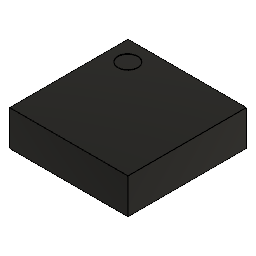
IMU v1 (Autodesk Fusion 360 design; units mm, degrees)
Autodesk Fusion 360 part; units mm, degrees
sketch "スケッチ1" plane through (0, 0, 0) normal (0, 0, 1) x (1, 0, 0)
  line L0 (1.5, 1.5) -> (-1.5, 1.5)
  line L1 (-1.5, 1.5) -> (-1.5, -1.5)
  line L2 (-1.5, -1.5) -> (1.5, -1.5)
  line L3 (1.5, -1.5) -> (1.5, 1.5)
  line L4 (1.5, 1.5) -> (-1.5, -1.5) construction
  line L5 (-1.5, 1.5) -> (1.5, -1.5) construction
  dimension "d1" = 3
  dimension "d2" = 3
extrude "押し出し1" add sketch "スケッチ1" along normal blind 0.9
sketch "スケッチ2" plane through (0, 0, 0.9) normal (0, 0, 1) x (-1, 0, 0)
  line L0 (-1.5, 1.5) -> (-1.5, -1.5)
  line L1 (-1.5, -1.5) -> (1.5, -1.5)
  line L2 (1.5, -1.5) -> (1.5, 1.5)
  line L3 (1.5, 1.5) -> (-1.5, 1.5)
  circle A0 centre (1.0021, -0.9978) radius 0.25
  dimension "d5" = 0.5
  measures "d5" diameter of A0
extrude "押し出し2" cut sketch "スケッチ2" against normal blind 0.01 contours A0
